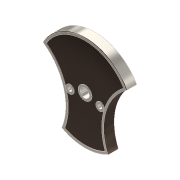
# Autodesk Inventor part: Disk
Saved by Autodesk Inventor 2022.2 (Build 262287010, 287A)
## iProperties
Created: 2022-12-22
Part Number: Disk
Material: Steel
Document SubType Name: Modeling
Designer: User
Mass: 335.354 g
Surface Area: 130.026 cm^2
Volume: 42.7203 cm^3
Density: 7.85 g/cm^3
Appearance: Gunmetal - Antique Polished
Author: User
Autodesk Inventor part; units mm, degrees
ref_plane "YZ Plane" through (0, 0, 0) normal (1, 0, 0) x (0, 1, 0)
ref_plane "XZ Plane" through (0, 0, 0) normal (0, 1, 0) x (-1, 0, 0)
ref_plane "XY Plane" through (0, 0, 0) normal (0, 0, 1) x (1, 0, 0)
sketch "Sketch1" plane through (0, 0, 0) normal (0, 0, 1) x (1, 0, 0)
  arc A0 (-44.218038, -12.679318) -> (-22.234092, -40.269655) centre (0, 0) ccw construction
  arc A1 (-22.234092, -40.269655) -> (-40.195246, 22.368331) centre (-70.172104, -20.121527) ccw
  line L0 (0, 0) -> (-70.172104, -20.121527) construction
  line L1 (0, -64.4) -> (0, 64.4) construction
  arc A2 (40.195246, 22.368331) -> (22.234092, -40.269655) centre (70.172104, -20.121527) ccw
  line L2 (0, 0) -> (70.172104, -20.121527) construction
  arc A3 (-40.195246, 22.368331) -> (-44.218038, 12.679318) centre (0, 0) ccw construction
  arc A4 (-22.234092, -40.269655) -> (22.234092, -40.269655) centre (0, 0) ccw
  arc A5 (22.234092, -40.269655) -> (40.195246, 22.368331) centre (0, 0) ccw construction
  arc A6 (40.195246, 22.368331) -> (-40.195246, 22.368331) centre (0, 0) ccw
  arc A7 (-44.218038, 12.679318) -> (-44.218038, -12.679318) centre (0, 0) ccw construction
  dimension "d0" = 92
  dimension "d1" = 52
  dimension "d2" = 73
  dimension "d3" = 148
  constraints: 16 point on circle, 8 centre point, 4 end point, 3 symmetric about line, 2 point on line, 1 coincident, 1 other
  measures "d0" diameter of A0
  measures "d1" radius of A1
  measures "d2" distance of L0.start L0.end
  measures "d3" angle of L2 L0
extrude "Extrusion1" add sketch "Sketch1" along normal mid plane 10
sketch "Sketch2" plane through (0, 0, 5) normal (0, 0, 1) x (1, 0, 0)
  arc A0 (-22.234092, -40.269655) -> (-40.195246, 22.368331) centre (-70.172104, -20.121527) ccw
  arc A1 (-22.234092, -40.269655) -> (22.234092, -40.269655) centre (0, 0) ccw
  arc A2 (40.195246, 22.368331) -> (22.234092, -40.269655) centre (70.172104, -20.121527) ccw
  arc A3 (40.195246, 22.368331) -> (-40.195246, 22.368331) centre (0, 0) ccw
  line L0 (0, 0) -> (-70.172104, -20.121527) construction
  line L1 (0, 0) -> (70.172104, -20.121527) construction
  point P0 (-14.418925, -4.13456)
  point P1 (14.418925, -4.13456)
  dimension "d6" = 15
  dimension "d7" = 15
  constraints: 4 end point, 2 point on line
  measures "d6" distance of point (-14.419, -4.135) A1.centre
  measures "d7" distance of point (14.419, -4.135) A1.centre
hole "Hole1" at (-14.418925, -4.13456, 5) at (14.418925, -4.13456, 5) direction (0, 0, -1) diameter 4 end through all
sketch "Sketch3" plane through (0, 0, 5) normal (0, 0, 1) x (1, 0, 0)
  arc A0 (-22.234092, -40.269655) -> (22.234092, -40.269655) centre (0, 0) ccw
hole "Hole2" at (0, 0, 5) direction (0, 0, -1) diameter 9 end through all
chamfer "Chamfer1" distance 0.5 angle 45 4 edges at (0, 46, 5) (0, 46, -5) (0, -46, -5) (0, -46, 5)
sketch "Sketch4" plane through (0, 0, 5) normal (0, 0, 1) x (1, 0, 0)
  arc A0 (-22.041384, -39.804866) -> (22.041384, -39.804866) centre (0, 0) ccw
  arc A1 (39.785519, 22.076287) -> (22.041384, -39.804866) centre (70.172104, -20.121527) ccw
  arc A2 (39.785519, 22.076287) -> (-39.785519, 22.076287) centre (0, 0) ccw
  arc A3 (-22.041384, -39.804866) -> (-39.785519, 22.076287) centre (-70.172104, -20.121527) ccw
  circle A4 centre (0, 0) radius 4.5
  circle A5 centre (-14.418925, -4.13456) radius 2
  circle A6 centre (14.418925, -4.13456) radius 2
  arc A7 (37.160523, 22.61295) -> (-37.160523, 22.61295) centre (0, 0) ccw
  arc A8 (37.160523, 22.61295) -> (19.530873, -38.868946) centre (70.172104, -20.121527) ccw
  arc A9 (-19.530873, -38.868946) -> (19.530873, -38.868946) centre (0, 0) ccw
  arc A10 (-19.530873, -38.868946) -> (-37.160523, 22.61295) centre (-70.172104, -20.121527) ccw
  circle A11 centre (-14.418925, -4.13456) radius 4
  circle A12 centre (0, 0) radius 6.5
  circle A13 centre (14.418925, -4.13456) radius 4
  dimension "d25" = 2
  dimension "d26" = 2
  dimension "d27" = 2
  dimension "d28" = 2
  constraints: 8 point on circle, 7 centre point, 3 other
  measures "d25" radial gap between concentric circles of A2 A7
  measures "d26" radial gap between concentric circles of A5 A11
  measures "d27" radial gap between concentric circles of A4 A12
  measures "d28" radial gap between concentric circles of A6 A13
extrude "Extrusion2" cut sketch "Sketch4" against normal blind 0.5 contours A8 A9 A10 A7
mirror "Mirror1" about plane through (0, 0, 0) normal (0, 0, 1) of "Extrusion2"
equation "\"d7\" = d6"
body "Solid1"
